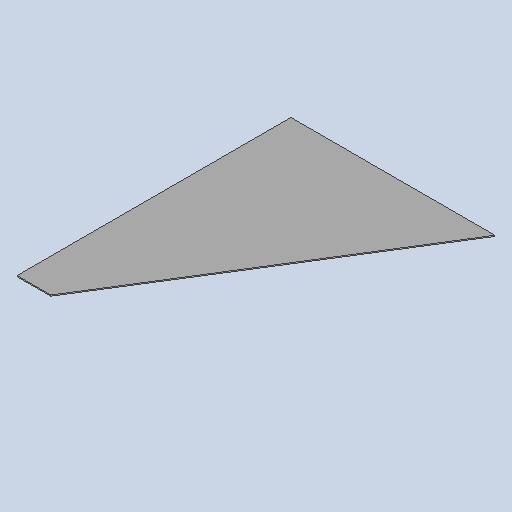
# Autodesk Inventor part: BSH 016 cone
Saved by Autodesk Inventor 2025 (Build 290162010, 162A)
## iProperties
Created: 2024-07-23
Part Number: BSH 016 cone
Material: 09g2s
Document SubType Name: Sheet Metal
Designer: admin
Mass: 76193.9 g
Surface Area: 64946.6 cm^2
Volume: 9706.23 cm^3
Density: 7.85 g/cm^3
Flat Pattern Width: 60.5 cm
Flat Pattern Length: 81.2 cm
Flat Pattern Area: 4912.6 cm^2
Sheet Metal Rule: AISI304 3mm Die 32
Sheet Metal Width: 605,000 mm
Sheet Metal Length: 812,000 mm
Sheet Metal Area: 491260,000 mm^2
Appearance: Default
Stock Number: БШК 016 конус
Author: admin
Autodesk Inventor part; units mm, degrees
ref_plane "YZ Plane" through (0, 0, 0) normal (1, 0, 0) x (0, 1, 0)
ref_plane "XZ Plane" through (0, 0, 0) normal (0, 1, 0) x (-1, 0, 0)
ref_plane "XY Plane" through (0, 0, 0) normal (0, 0, 1) x (1, 0, 0)
sketch "Sketch5" plane through (0, 0, 0) normal (0, 0, 1) x (1, 0, 0)
  line L0 (0, 0) -> (100, 0)
  line L1 (100, 0) -> (605, 812)
  line L2 (605, 812) -> (0, 812)
  line L3 (0, 812) -> (0, 0)
  dimension "d37" = 100
  dimension "d38" = 812
  dimension "d39" = 605
  measures "d37" distance of L0.start L0.end
  measures "d38" distance of L2.end L0.start
  measures "d39" distance of L1.end L2.end
extrude "Plate4" add sketch "Sketch5" along normal blind 3
equation "\"d28\" = Thickness"
equation "\"BendReliefWidth\" = Thickness"
equation "\"BendReliefDepth\" = 0.5 * Thickness"
equation "\"CornerReliefSize\" = 4 * Thickness"
equation "\"MinimumRemnant\" = 2 * Thickness"
equation "\"TransitionRadius\" = BendRadius"
equation "\"JacobiRadiusSize\" = BendRadius"
equation "\"GapSize\" = Thickness"
equation "\"Thickness\" = 3"
equation "\"BendRadius\" = 5"
body "Solid2"
